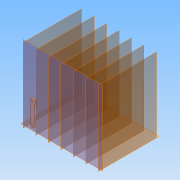
# Autodesk Inventor part: Selection_Ramp 1_LHS piece
Saved by Autodesk Inventor 2018.1 (Build 221171000, 171)
## iProperties
Created: 2019-02-07
Part Number: Selection_Ramp 1_LHS piece
Material: Wood (Cherry)
Document SubType Name: Modeling
Designer: James
Density: 0.63 g/cm^3
Appearance: Cherry - Natural Low Gloss
Author: James
Autodesk Inventor part; units mm, degrees
ref_plane "YZ Plane" through (0, 0, 0) normal (1, 0, 0) x (0, 1, 0)
ref_plane "XZ Plane" through (0, 0, 0) normal (0, 1, 0) x (-1, 0, 0)
ref_plane "XY Plane" through (0, 0, 0) normal (0, 0, 1) x (1, 0, 0)
derived "Selection_Skeleton.ipt"
ref_plane "Ground" through (0, 0, 0) normal (0, 1, 0) x (-1, 0, 0)
ref_plane "LHS inner" through (0, 0, 0) normal (1, 0, 0) x (0, 1, 0)
ref_plane "RHS inner" through (300, 0, 0) normal (1, 0, 0) x (0, 1, 0)
ref_plane "Lane 1" through (50, 0, 0) normal (1, 0, 0) x (0, 1, 0)
ref_plane "Lane 2" through (100, 0, 0) normal (1, 0, 0) x (0, 1, 0)
ref_plane "Lane 3" through (150, 0, 0) normal (1, 0, 0) x (0, 1, 0)
ref_plane "Lane 4" through (200, 0, 0) normal (1, 0, 0) x (0, 1, 0)
ref_plane "Lane 5" through (250, 0, 0) normal (1, 0, 0) x (0, 1, 0)
ref_plane "Back" through (0, 0, 0) normal (0, 0, 1) x (1, 0, 0)
sketch "Sketch1" plane through (0, 0, 0) normal (0, 1, 0) x (-1, 0, 0)
  line L0 (-20, 0) -> (-20, 100)
  line L1 (-20, 100) -> (-37.5, 100)
  line L2 (-37.5, 100) -> (-32.5, 0)
  line L3 (-32.5, 0) -> (-20, 0)
  line L4 (-50, -20) -> (-50, 120) projected
  line L5 (-100, -20) -> (-100, 120) projected
  line L6 (-45, 0) -> (7.5, 0) projected
  point P0 (0, 0)
  dimension "d1" = 100
  dimension "d21" = 17.5
  dimension "d22" = 12.5
  dimension "d23" = 12.5
  constraints: 8 end point, 1 collinear, 1 horizontal, 1 parallel, 1 vertical alignment
  measures "d1" distance between parallel lines of L3 L1
  measures "d21" distance from line of L4 L2.end
  measures "d22" distance from line of L4 L1.end
  measures "d23" distance of L2.end L0.start
extrude "Extrusion1" add sketch "Sketch1" along normal blind 5
sketch "Sketch2" plane through (0, 5, 0) normal (0, 1, 0) x (1, 0, 0)
  line L0 (20, -100) -> (37.5, -100) projected
  line L1 (32.5, 0) -> (20, 0) projected
  line L2 (20, 0) -> (20, -100) projected
  point P0 (0, 0)
  point P1 (25, -10)
  point P2 (25, -90)
  dimension "d9" = 10
  dimension "d10" = 10
  dimension "d11" = 80
  dimension "d24" = 5
  constraints: 1 vertical alignment
  measures "d9" distance from line of L0 point (25, -90)
  measures "d10" distance from line of point (25, -10) L1
  measures "d11" distance of point (25, -90) point (25, -10)
  measures "d24" distance from line of L2 point (25, -10)
hole "Hole1" at (25, 5, 10) at (25, 5, 90) direction (0, -1, 0) diameter 4.5 end through all countersink diameter 9.4 countersink angle 90 clearance for "Flat Head Machine Screw" size "M4" standard "Ansi Metric M Profile"
equation "\"d10\" = d9"
body "Solid1"
